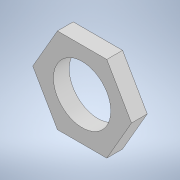
# Autodesk Inventor part: DC Jack Nut
Saved by Autodesk Inventor 2022 (Build 260153000, 153)
## iProperties
Created: 2022-06-10
Part Number: DC Jack Nut
Material: Generic
Document SubType Name: Modeling
Designer: Nick
Density: 1 g/cm^3
Appearance: Default
Author: Nick
Autodesk Inventor part; units mm, degrees
ref_plane "YZ Plane" through (0, 0, 0) normal (1, 0, 0) x (0, 1, 0)
ref_plane "XZ Plane" through (0, 0, 0) normal (0, 1, 0) x (-1, 0, 0)
ref_plane "XY Plane" through (0, 0, 0) normal (0, 0, 1) x (1, 0, 0)
sketch "Sketch1" plane through (0, 0, 0) normal (0, 0, 1) x (1, 0, 0)
  line L0 (6.2643, 0) -> (3.1321, -5.425)
  line L1 (3.1321, -5.425) -> (-3.1321, -5.425)
  line L2 (-3.1321, -5.425) -> (-6.2643, 0)
  line L3 (-6.2643, 0) -> (-3.1321, 5.425)
  line L4 (-3.1321, 5.425) -> (3.1321, 5.425)
  line L5 (3.1321, 5.425) -> (6.2643, 0)
  circle A0 centre (0, 0) radius 3.64
  dimension "d0" = 10.85
  dimension "d1" = 7.28
  constraints: 12 end point, 2 coincident, 1 centre point, 1 horizontal, 13 other
  measures "d0" distance between parallel lines of L1 L4
  measures "d1" diameter of A0
extrude "Extrusion1" add sketch "Sketch1" along normal blind 2
body "Solid1"
